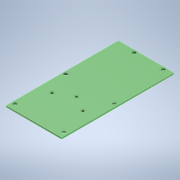
# Autodesk Inventor part: EChem Sensor Board Lower
Saved by Autodesk Inventor 2021 (Build 250183000, 183)
## iProperties
Created: 2020-07-06
Part Number: EChem Sensor Board Lower
Material: Generic
Document SubType Name: Modeling
Designer: jgray
Density: 1 g/cm^3
Appearance: Default
Author: jgray
Autodesk Inventor part; units mm, degrees
ref_plane "YZ Plane" through (0, 0, 0) normal (1, 0, 0) x (0, 1, 0)
ref_plane "XZ Plane" through (0, 0, 0) normal (0, 1, 0) x (-1, 0, 0)
ref_plane "XY Plane" through (0, 0, 0) normal (0, 0, 1) x (1, 0, 0)
sketch "Sketch1" plane through (0, 0, 0) normal (0, 1, 0) x (-1, 0, 0)
  line L0 (0, 0) -> (53.34, 0)
  line L1 (53.34, 0) -> (53.34, -107.95)
  line L2 (53.34, -107.95) -> (0, -107.95)
  line L3 (0, -107.95) -> (0, 0)
  point P0 (50.34, -5.5)
  point P1 (3.34, -5.5)
  point P2 (50.7579, -54.61)
  point P3 (2.8578, -53.34)
  point P4 (35.56, -105.41)
  point P5 (7.62, -105.41)
  dimension "d0" = 53.34
  dimension "d1" = 107.95
  dimension "d2" = 3
  dimension "d3" = 5.5
  dimension "d4" = 5.5
  dimension "d5" = 3.34
  dimension "d6" = 53.34
  dimension "d7" = 54.61
  dimension "d8" = 2.54
  dimension "d9" = 2.54
  dimension "d10" = 7.62
  dimension "d11" = 17.78
  constraints: 8 end point, 2 parallel, 1 horizontal, 1 perpendicular
  measures "d0" distance of L1.end L2.end
  measures "d1" distance of L0.end L1.end
  measures "d2" distance from line of L1 point (50.34, -5.5)
  measures "d3" distance from line of L0 point (50.34, -5.5)
  measures "d4" vertical distance of L0.start point (3.34, -5.5)
  measures "d5" distance from line of L3 point (3.34, -5.5)
  measures "d6" distance from line of point (2.858, -53.34) L0
  measures "d7" distance from line of L0 point (50.758, -54.61)
  measures "d8" distance from line of L2 point (35.56, -105.41)
  measures "d9" distance from line of L2 point (7.62, -105.41)
  measures "d10" distance from line of L3 point (7.62, -105.41)
  measures "d11" distance from line of L1 point (35.56, -105.41)
extrude "Extrusion1" add sketch "Sketch1" against normal blind 1.65
hole "Hole1" at (-50.34, 0, -5.5) at (-3.34, 0, -5.5) at (-50.7579, 0, -54.61) at (-2.8578, 0, -53.34) at (-35.56, 0, -105.41) at (-7.62, 0, -105.41) direction (0, -1, 0) diameter 3.2 end through all
sketch "Sketch2" plane through (0, 0, 0) normal (0, 1, 0) x (1, 0, 0)
  line L0 (-53.34, 0) -> (0, 0) projected
  line L1 (0, 0) -> (0, 107.95) projected
  circle A0 centre (-26.67, 23.67) radius 17.2
  line L2 (-26.67, 23.67) -> (-26.67, 130.1739)
  line L3 (-26.67, 23.67) -> (-67.3773, 47.1724)
  line L4 (-26.67, 23.67) -> (20.3348, 23.67) construction
  line L5 (-26.67, 23.67) -> (24.306, 53.101)
  line L6 (-26.67, 23.67) -> (32.192, 23.67) construction
  point P0 (-26.67, 40.87)
  point P1 (-11.7744, 32.27)
  point P2 (-26.67, 40.87)
  point P3 (-41.5656, 32.27)
  dimension "d21" = 23.67
  dimension "d22" = 26.67
  dimension "d23" = 34.4
  dimension "d24" = 150
  dimension "d25" = 30
  constraints: 10 end point, 3 point on circle, 3 point on line, 2 coincident, 2 equal length, 2 horizontal, 1 centre point, 1 vertical
  measures "d21" distance from line of point (-26.67, 23.67) L0
  measures "d22" distance from line of point (-26.67, 23.67) L1
  measures "d23" diameter of A0
  measures "d24" angle of L4 L3
  measures "d25" angle of L6 L5
hole "Hole2" at (-26.67, 0, -40.87) at (-11.7744, 0, -32.27) at (-41.5656, 0, -32.27) direction (0, -1, 0) diameter 2.58 end through all
body "Solid1"
